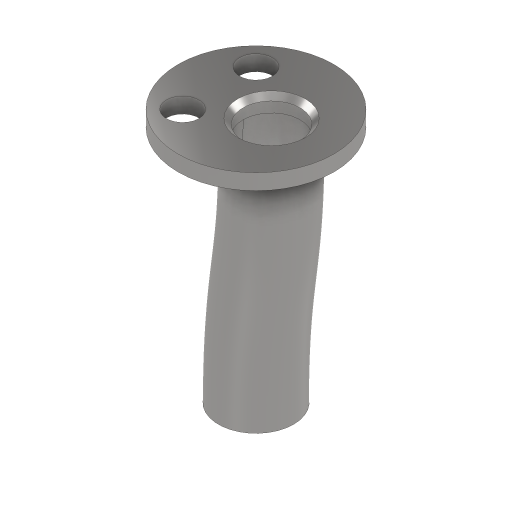
# Autodesk Inventor part: Nipple-3dprinted-metal
Saved by Autodesk Inventor 2024.2 (Build 282272000, 272)
## iProperties
Created: 2024-02-08
Part Number: Nipple-3dprinted-metal
Material: Stainless Steel
Document SubType Name: Modeling
Designer: kuzmin
Density: 8 g/cm^3
Appearance: Semi-Polished
Author: kuzmin
Autodesk Inventor part; units mm, degrees
ref_plane "YZ Plane" through (0, 0, 0) normal (1, 0, 0) x (0, 1, 0)
ref_plane "XZ Plane" through (0, 0, 0) normal (0, 1, 0) x (-1, 0, 0)
ref_plane "XY Plane" through (0, 0, 0) normal (0, 0, 1) x (1, 0, 0)
sketch "Sketch1" plane through (0, 0, 0) normal (0, 1, 0) x (-1, 0, 0)
  circle A0 centre (0, 0) radius 7.25
  circle A1 centre (0, 0) radius 5.5
  dimension "d0" = 14.5
  dimension "d7" = 11
  constraints: 2 centre point, 2 coincident
  measures "d0" diameter of A0
  measures "d7" diameter of A1
sketch "Sketch2" plane through (0, 0, 0) normal (0, 0, 1) x (1, 0, 0)
  line L0 (0, 0) -> (0, 23) construction
  line L1 (0, 23) -> (3, 23) construction
  line L2 (3, 23) -> (3, 46) construction
  spline S0 degree 3 poles (0, 0) (0, 23) (3, 23) (3, 46) knots 1 1 1 1 2 2 2 2
  line L3 (0, 46) -> (0, 0) construction
  line L4 (0, 46) -> (3, 46) construction
  dimension "d1" = 46
  dimension "d3" = 3
  constraints: 4 end point, 2 horizontal, 1 coincident, 1 midpoint, 1 parallel, 1 vertical, 3 other
  measures "d1" vertical distance of L0.start L2.end
  measures "d3" distance of L2.end L3.start
sweep "Sweep1" add profiles "Sketch1" path "Sketch2"
sketch "Sketch3" plane through (3, 46, 0) normal (0, 1, 0) x (1, 0, 0)
  circle A0 centre (-3, 0) radius 15
  circle A1 centre (-10.0711, 7.0711) radius 3.135
  circle A2 centre (-10.0711, -7.0711) radius 3.135
  circle A3 centre (-3, 0) radius 7.25 construction
  line L0 (-10.0711, 7.0711) -> (-3, 0) construction
  line L1 (-3, 0) -> (-18, 0) construction
  line L2 (-3, 0) -> (-10.0711, -7.0711) construction
  circle A4 centre (0, 0) radius 5.5 projected
  point P0 (-10.25, 0)
  point P1 (-5.5, 0)
  dimension "d8" = 30
  dimension "d9" = 6.27
  dimension "d10" = 45
  dimension "d11" = 45
  dimension "d12" = 10
  constraints: 6 end point, 3 horizontal alignment, 2 centre point, 2 coincident, 1 equal radius, 1 horizontal, 1 perpendicular, 2 other
  measures "d9" diameter of A1
  measures "d10" angle of L1 L0
  measures "d11" angle of L2 L1
  measures "d12" distance of L0.start L0.end
extrude "Extrusion1" add sketch "Sketch3" along normal blind 3
chamfer "Chamfer1" distance 1 angle 45 1 edges at (10.25, 46, 0)
chamfer "Chamfer2" distance 1 angle 45 1 edges at (-2.5, 49, 0)
body "Solid1"
